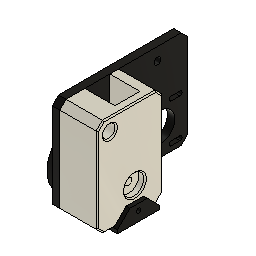
V2 Z Gearbox Buddy A (Autodesk Fusion 360 design; units mm, degrees)
Autodesk Fusion 360 part; units mm, degrees
sketch "Sketch1" plane through (0, 0, 0) normal (1, 0, 0) x (0, 1, 0)
  line L0 (21, 21) -> (-21, 21) construction
  line L1 (-21, 21) -> (-21, -21) construction
  line L2 (-21, -21) -> (21, -21) construction
  line L3 (21, -21) -> (21, 21) construction
  line L4 (21, 21) -> (-21, -21) construction
  line L5 (-21, 21) -> (21, -21) construction
  line L6 (15.5, 15.5) -> (-15.5, 15.5) construction
  line L7 (-15.5, 15.5) -> (-15.5, -15.5) construction
  line L8 (-15.5, -15.5) -> (15.5, -15.5) construction
  line L9 (15.5, -15.5) -> (15.5, 15.5) construction
  line L10 (15.5, 15.5) -> (-15.5, -15.5) construction
  line L11 (-15.5, 15.5) -> (15.5, -15.5) construction
  line L12 (21, -21) -> (-77, -21)
  line L13 (-77, -21) -> (-77, 57)
  line L14 (-77, 57) -> (21, 57)
  line L15 (21, 57) -> (21, -21) construction
  circle A0 centre (0, 0) radius 8 construction
  circle A1 centre (0, 0) radius 6.11 construction
  line L16 (-77, 37) -> (25, 37)
  line L17 (-77, 32) -> (25, 32)
  circle A2 centre (-47, 0) radius 30 construction
  circle A3 centre (0, 0) radius 2.75
  circle A4 centre (-47, 0) radius 2.75
  line L18 (-47, 37) -> (-47, 32)
  line L19 (19, 17.2) -> (12, 17.2)
  arc A5 (12, 17.2) -> (12, 13.8) centre (12, 15.5) ccw
  line L20 (12, 13.8) -> (19, 13.8)
  arc A6 (19, 13.8) -> (19, 17.2) centre (19, 15.5) ccw
  line L21 (19, 15.5) -> (12, 15.5) construction
  line L22 (-12, 17.2) -> (-19, 17.2)
  arc A7 (-19, 17.2) -> (-19, 13.8) centre (-19, 15.5) ccw
  arc A8 (-12, 13.8) -> (-12, 17.2) centre (-12, 15.5) ccw
  line L23 (-19, 13.8) -> (-12, 13.8)
  line L24 (19, -13.8) -> (12, -13.8)
  arc A9 (12, -13.8) -> (12, -17.2) centre (12, -15.5) ccw
  arc A10 (19, -17.2) -> (19, -13.8) centre (19, -15.5) ccw
  line L25 (12, -17.2) -> (19, -17.2)
  line L26 (-12, -13.8) -> (-19, -13.8)
  arc A11 (-19, -13.8) -> (-19, -17.2) centre (-19, -15.5) ccw
  arc A12 (-12, -17.2) -> (-12, -13.8) centre (-12, -15.5) ccw
  line L27 (-19, -17.2) -> (-12, -17.2)
  line L28 (21, 57) -> (25, 57)
  line L29 (25, 57) -> (25, -21)
  line L30 (25, -21) -> (21, -21)
  line L31 (21, -21) -> (21, 57) construction
  line L32 (-47, -21) -> (-47, 0) construction
  line L33 (-47, 0) -> (-77, 0) construction
  line L34 (0, 0) -> (-47, 0) construction
  point P0 (15.5, 15.5)
  dimension "d488" = 42
  dimension "d489" = 42
  dimension "d490" = 31
  dimension "d491" = 31
  dimension "d492" = 16
  dimension "d493" = 12.22
  dimension "d494" = 20
  dimension "d496" = 60
  dimension "d498" = 98
  dimension "d499" = 78
  dimension "d502" = 5.5
  dimension "d503" = 5.5
  dimension "d506" = 30
  dimension "d507" = 3.4
  dimension "d508" = 7
  dimension "d511" = -31
  dimension "d512" = -31
  dimension "d513" = 4
  dimension "d5757" = 30
  dimension "d5758" = 21
  dimension "d5762" = 102
  dimension "d5763" = 47
  constraint horizontal L0
  constraint perpendicular L0 L1
  constraint parallel L0 L2
  constraint parallel L1 L3
  constraint coincident L4 A0.centre
  constraint coincident L5 A0.centre
  constraint coincident A0.centre A1.centre
  constraint horizontal L6
  constraint perpendicular L6 L7
  constraint parallel L6 L8
  constraint parallel L7 L9
  constraint coincident L10 A0.centre
  constraint coincident L11 A0.centre
  constraint horizontal L12
  constraint vertical L13
  constraint horizontal L14
  constraint vertical L15
  constraint coincident L2.end L12
  constraint coincident L0.start L15
  constraint coincident L13 L16.start
  constraint perpendicular L13 L16
  constraint coincident L13 L17.start
  constraint concentric A2 A4
  constraint coincident L16 L18.start
  constraint coincident L17 L18.end
  constraint perpendicular L17 L18
  constraint tangent L19 A5
  constraint tangent A5 L20
  constraint parallel L19 L20
  constraint tangent L20 A6
  constraint tangent L19 A6
  constraint coincident L6 A5.centre
  constraint perpendicular L9 L21
  constraint coincident P0 L6.start
  constraint midpoint L21 P0
  constraint horizontal L28
  constraint vertical L29
  constraint horizontal L30
  constraint vertical L31
  constraint coincident L2.end L3.start
  constraint coincident L29 L16.end
  constraint coincident L29 L17.end
  constraint coincident L12 L32.start
  constraint perpendicular L12 L32
  constraint perpendicular L13 L33
  constraint coincident L13 L33.end
  constraint coincident A2.centre A4.centre
  measures "d488" distance of L0.start L2.end
  measures "d489" distance of L0.start L0.end
  measures "d490" distance of L7.end L8.end
  measures "d491" distance of L6.end L7.end
  measures "d492" diameter of A0
  measures "d493" diameter of A1
  measures "d494" distance of L14 L16
  measures "d496" diameter of A2
  measures "d498" distance of L2.end L12.end
  measures "d499" distance of L12.end L13.end
  measures "d502" diameter of A3
  measures "d503" diameter of A4
  measures "d506" distance of L13 L18
  measures "d507" diameter of A5
  measures "d508" distance of A6.centre A5.centre
  measures "d513" distance of L29.end L2.end
  measures "d5757" distance of L13 L32
  measures "d5758" distance of L12 L33
  measures "d5762" distance of L13 L29
  measures "d5763" distance of A2.centre A0.centre
extrude "Extrude1" add sketch "Sketch1" along normal blind 6 makes body 1
extrude "Extrude2" add sketch "Sketch1" against normal blind 20 contours L16 L17 L18 L29 bodies 1
sketch "Sketch2" plane through (0, 0, 0) normal (-1, 0, 0) x (0, -1, 0)
  line L0 (-25, 37) -> (47, 37)
  line L1 (47, 37) -> (47, 32)
  line L2 (47, 32) -> (-25, 32)
  line L3 (-25, 32) -> (-25, -21)
  line L4 (-25, -21) -> (77, -21)
  line L5 (77, -21) -> (77, 57)
  line L6 (77, 57) -> (-25, 57)
  line L7 (-25, 57) -> (-25, 37)
  line L8 (-12, -17.2) -> (-19, -17.2)
  arc A0 (-19, -13.8) -> (-19, -17.2) centre (-19, -15.5) ccw
  line L9 (-19, -13.8) -> (-12, -13.8)
  arc A1 (-12, -17.2) -> (-12, -13.8) centre (-12, -15.5) ccw
  arc A2 (-19, 17.2) -> (-19, 13.8) centre (-19, 15.5) ccw
  line L10 (-19, 17.2) -> (-12, 17.2)
  arc A3 (-12, 13.8) -> (-12, 17.2) centre (-12, 15.5) ccw
  line L11 (-12, 13.8) -> (-19, 13.8)
  line L12 (19, -17.2) -> (12, -17.2)
  arc A4 (12, -13.8) -> (12, -17.2) centre (12, -15.5) ccw
  line L13 (12, -13.8) -> (19, -13.8)
  arc A5 (19, -17.2) -> (19, -13.8) centre (19, -15.5) ccw
  line L14 (19, 13.8) -> (12, 13.8)
  arc A6 (12, 17.2) -> (12, 13.8) centre (12, 15.5) ccw
  line L15 (12, 17.2) -> (19, 17.2)
  arc A7 (19, 13.8) -> (19, 17.2) centre (19, 15.5) ccw
  circle A8 centre (47, 0) radius 2.75
  circle A9 centre (0, 0) radius 2.75
  line L16 (-3.5, -11.5) -> (3.5, -11.5)
  arc A10 (3.5, -11.5) -> (3.5, 11.5) centre (3.5, 0) ccw
  line L17 (3.5, 11.5) -> (-3.5, 11.5)
  arc A11 (-3.5, 11.5) -> (-3.5, -11.5) centre (-3.5, 0) ccw
  line L18 (-3.5, 0) -> (3.5, 0) construction
  line L19 (15.5, -15.5) -> (-15.5, -15.5) construction
  line L20 (-15.5, -15.5) -> (-15.5, 15.5) construction
  line L21 (-15.5, 15.5) -> (15.5, 15.5) construction
  line L22 (15.5, 15.5) -> (15.5, -15.5) construction
  line L23 (15.5, -15.5) -> (-15.5, 15.5) construction
  line L24 (-15.5, -15.5) -> (15.5, 15.5) construction
  line L25 (-18.5, 11.5) -> (-12.5, 11.5)
  arc A12 (-12.5, 11.5) -> (-12.5, 19.5) centre (-12.5, 15.5) ccw
  line L26 (-12.5, 19.5) -> (-18.5, 19.5)
  arc A13 (-18.5, 19.5) -> (-18.5, 11.5) centre (-18.5, 15.5) ccw
  line L27 (-18.5, 15.5) -> (-12.5, 15.5) construction
  line L28 (18.5, 19.5) -> (12.5, 19.5)
  arc A14 (12.5, 19.5) -> (12.5, 11.5) centre (12.5, 15.5) ccw
  arc A15 (18.5, 11.5) -> (18.5, 19.5) centre (18.5, 15.5) ccw
  line L29 (12.5, 11.5) -> (18.5, 11.5)
  line L30 (-12.5, -11.5) -> (-18.5, -11.5)
  arc A16 (-18.5, -11.5) -> (-18.5, -19.5) centre (-18.5, -15.5) ccw
  arc A17 (-12.5, -19.5) -> (-12.5, -11.5) centre (-12.5, -15.5) ccw
  line L31 (-18.5, -19.5) -> (-12.5, -19.5)
  line L32 (18.5, -11.5) -> (12.5, -11.5)
  arc A18 (12.5, -11.5) -> (12.5, -19.5) centre (12.5, -15.5) ccw
  arc A19 (18.5, -19.5) -> (18.5, -11.5) centre (18.5, -15.5) ccw
  line L33 (12.5, -19.5) -> (18.5, -19.5)
  point P0 (-15.5, 15.5)
  dimension "d514" = 23
  dimension "d515" = 7
  dimension "d556" = 31
  dimension "d557" = 31
  dimension "d558" = 4
  dimension "d559" = 6
  dimension "d562" = 31
  dimension "d563" = -31
  constraint tangent L16 A10
  constraint tangent A10 L17
  constraint parallel L16 L17
  constraint tangent L17 A11
  constraint tangent L16 A11
  constraint perpendicular L3 L18
  constraint coincident A9.centre origin
  constraint midpoint L18 A9.centre
  constraint horizontal L19
  constraint perpendicular L19 L20
  constraint parallel L19 L21
  constraint parallel L20 L22
  constraint coincident L23 A9.centre
  constraint coincident L24 A9.centre
  constraint tangent L25 A12
  constraint tangent A12 L26
  constraint parallel L25 L26
  constraint tangent L26 A13
  constraint tangent L25 A13
  constraint coincident L21 A12.centre
  constraint perpendicular L20 L27
  constraint coincident P0 L20.end
  constraint midpoint L27 P0
  measures "d514" diameter of A10
  measures "d515" distance of A11.centre A10.centre
  measures "d556" distance of P0 L21.end
  measures "d557" distance of L19.end P0
  measures "d558" radius of A12
  measures "d559" distance of A13.centre A12.centre
extrude "Extrude3" cut sketch "Sketch2" against normal through all contours L16 A10 L17 A11 bodies 1
extrude "Extrude4" cut sketch "Sketch2" against normal blind 1.5 contours L25 A12 L26 A13 | L28 A14 A15 L29 | L30 A16 A17 L31 | L32 A18 A19 L33 bodies 1
hole "Hole1" at (-10, -11, 37) direction (0, 0, -1) diameter 5.5 end through all bodies 1
sketch "Sketch3" plane through (0, 0, 0) normal (-1, 0, 0) x (0, -1, 0)
  line L0 (-3.5, 11.5) -> (3.5, 11.5)
  arc A0 (3.5, -11.5) -> (3.5, 11.5) centre (3.5, 0) ccw
  line L1 (3.5, -11.5) -> (-3.5, -11.5)
  arc A1 (-3.5, 11.5) -> (-3.5, -11.5) centre (-3.5, 0) ccw
  line L2 (-25, 37) -> (47, 37)
  line L3 (47, 37) -> (47, 32)
  line L4 (47, 32) -> (-25, 32)
  line L5 (-25, 32) -> (-25, -21)
  line L6 (-25, -21) -> (77, -21)
  line L7 (77, -21) -> (77, 57)
  line L8 (77, 57) -> (-25, 57)
  line L9 (-25, 57) -> (-25, 37)
  circle A2 centre (47, 0) radius 2.75
  line L10 (-25, 57) -> (-25, 37)
  line L11 (-25, 47) -> (-1, 47) construction
  arc A3 (18.5, 11.5) -> (18.5, 19.5) centre (18.5, 15.5) ccw
  line L12 (18.5, 11.5) -> (12.5, 11.5)
  arc A4 (12.5, 19.5) -> (12.5, 11.5) centre (12.5, 15.5) ccw
  line L13 (12.5, 19.5) -> (18.5, 19.5)
  arc A5 (18.5, -19.5) -> (18.5, -11.5) centre (18.5, -15.5) ccw
  line L14 (18.5, -19.5) -> (12.5, -19.5)
  arc A6 (12.5, -11.5) -> (12.5, -19.5) centre (12.5, -15.5) ccw
  line L15 (12.5, -11.5) -> (18.5, -11.5)
  line L16 (-12.5, 11.5) -> (-18.5, 11.5)
  arc A7 (-18.5, 19.5) -> (-18.5, 11.5) centre (-18.5, 15.5) ccw
  line L17 (-18.5, 19.5) -> (-12.5, 19.5)
  arc A8 (-12.5, 11.5) -> (-12.5, 19.5) centre (-12.5, 15.5) ccw
  arc A9 (-12.5, -19.5) -> (-12.5, -11.5) centre (-12.5, -15.5) ccw
  line L18 (-12.5, -19.5) -> (-18.5, -19.5)
  arc A10 (-18.5, -11.5) -> (-18.5, -19.5) centre (-18.5, -15.5) ccw
  line L19 (-18.5, -11.5) -> (-12.5, -11.5)
  dimension "d549" = 24
  constraint midpoint L10 L11.start
  constraint perpendicular L10 L11
  measures "d549" distance of L11.start L11.end
hole "Hole3" at (0, 1, 47) direction (1, 0, 0) diameter 5.5 end through all bodies 1
hole "Hole4" at (0, -47, 0) direction (1, 0, 0) diameter 16.2 depth 5 tip angle 180 bodies 1
chamfer "Chamfer1" distance 20 angle 45 2 edges at (-20, 25, 34.5) (-20, -47, 34.5) on bodies 1
chamfer "Chamfer2" distance 5 angle 45 4 edges at (3, -77, 57) (3, -77, -21) (3, 25, -21) (3, 25, 57) on bodies 1
chamfer "Chamfer3" distance 0.5 angle 45 1 edges at (0, -39.4481, 2.9291) on bodies 1
sketch "Sketch1 (2)" plane through (6, 0, 0) normal (1, 0, 0) x (0, 1, 0) in component "V2 Z Gearbox Cover A"
  line L0 (25, 52) -> (20, 57)
  line L1 (20, 57) -> (-72, 57)
  line L2 (-72, 57) -> (-77, 52)
  line L3 (-77, 52) -> (-77, -16)
  line L4 (-77, -16) -> (-72, -21)
  line L5 (-72, -21) -> (20, -21)
  line L6 (20, -21) -> (25, -16)
  line L7 (25, -16) -> (25, 52)
  line L8 (-3.5, 11.5) -> (3.5, 11.5)
  arc A0 (3.5, -11.5) -> (3.5, 11.5) centre (3.5, 0) ccw
  line L9 (3.5, -11.5) -> (-3.5, -11.5)
  arc A1 (-3.5, 11.5) -> (-3.5, -11.5) centre (-3.5, 0) ccw
  line L10 (19, -17.2) -> (12, -17.2)
  arc A2 (12, -13.8) -> (12, -17.2) centre (12, -15.5) ccw
  line L11 (12, -13.8) -> (19, -13.8)
  arc A3 (19, -17.2) -> (19, -13.8) centre (19, -15.5) ccw
  line L12 (-12, -17.2) -> (-19, -17.2)
  arc A4 (-19, -13.8) -> (-19, -17.2) centre (-19, -15.5) ccw
  line L13 (-19, -13.8) -> (-12, -13.8)
  arc A5 (-12, -17.2) -> (-12, -13.8) centre (-12, -15.5) ccw
  circle A6 centre (-47, 0) radius 2.75
  arc A7 (19, 13.8) -> (19, 17.2) centre (19, 15.5) ccw
  line L14 (19, 13.8) -> (12, 13.8)
  arc A8 (12, 17.2) -> (12, 13.8) centre (12, 15.5) ccw
  line L15 (12, 17.2) -> (19, 17.2)
  line L16 (-12, 13.8) -> (-19, 13.8)
  arc A9 (-19, 17.2) -> (-19, 13.8) centre (-19, 15.5) ccw
  line L17 (-19, 17.2) -> (-12, 17.2)
  arc A10 (-12, 13.8) -> (-12, 17.2) centre (-12, 15.5) ccw
  circle A11 centre (-47, 0) radius 2.75
  line L18 (-47, 0) -> (-47, 57) construction
  line L19 (-47, 32) -> (25, 32)
  line L20 (21, -21) -> (-21, -21) construction
  line L21 (-21, -21) -> (-21, 21) construction
  line L22 (-21, 21) -> (21, 21) construction
  line L23 (21, 21) -> (21, -21) construction
  line L24 (21, -21) -> (-21, 21) construction
  line L25 (-21, -21) -> (21, 21) construction
  line L26 (-69, 57) -> (-25, 57)
  line L27 (-25, 57) -> (-25, -21)
  line L28 (-25, -21) -> (-69, -21)
  line L29 (-69, -21) -> (-69, 57)
  circle A12 centre (1, 47) radius 2.75
  point P0 (-47, 57)
  dimension "d521" = 42
  dimension "d522" = 42
  dimension "d524" = 44
  dimension "d525" = 4
  constraint coincident A6.centre A11.centre
  constraint perpendicular L1 L18
  constraint coincident P0 L18.end
  constraint horizontal L20
  constraint perpendicular L20 L21
  constraint parallel L20 L22
  constraint parallel L21 L23
  constraint coincident L24 origin
  constraint coincident L25 origin
  constraint horizontal L26
  constraint vertical L27
  constraint horizontal L28
  constraint vertical L29
  constraint coincident L5 L27.end
  constraint midpoint P0 L26
  constraint coincident L1 L26.start
  measures "d521" distance of L21.end L22.end
  measures "d522" distance of L20.end L21.end
  measures "d524" distance of L27.end L28.end
  measures "d525" distance of L21 L27
extrude "Extrude1'" add sketch "Sketch1 (2)" along normal blind 30 separate body contours L1 L5 L26 L27 L28 L29 makes body 2 in component "V2 Z Gearbox Cover A"
sketch "Sketch2 (2)" plane through (0, 0, 57) normal (0, 0, 1) x (-1, 0, 0) in component "V2 Z Gearbox Cover A"
  line L0 (-36, 44.25) -> (-36, 49.75)
  line L1 (-6, 44.25) -> (-6, 49.75)
  line L2 (-6, 47) -> (-18, 47) construction
  line L3 (-6, 57) -> (-30, 57)
  line L4 (-30, 57) -> (-30, 37)
  line L5 (-30, 37) -> (-6, 37)
  line L6 (-6, 37) -> (-6, 57)
  line L7 (-6, 57) -> (-30, 37) construction
  line L8 (-30, 57) -> (-6, 37) construction
  line L9 (-6, 69) -> (-6, 25)
  point P0 (-18, 47)
  dimension "d528" = 20
  dimension "d529" = 24
  dimension "d530" = 6
  constraint midpoint L1 L2.start
  constraint perpendicular L1 L2
  constraint horizontal L3
  constraint perpendicular L3 L4
  constraint parallel L3 L5
  constraint parallel L4 L6
  constraint coincident L7 P0
  constraint coincident L8 P0
  constraint coincident P0 L2.end
  constraint coincident L3.start L9
  measures "d528" distance of L3.end L4.end
  measures "d529" distance of L4 L6
  measures "d530" distance of L0 L4
extrude "Extrude2'" cut sketch "Sketch2 (2)" against normal through all bodies 2 in component "V2 Z Gearbox Cover A"
extrude "Extrude3'" add 1 faces at (16, -69, 5) along direction (0, -1, 0) up to surface (8 mm away) on bodies 2 bodies 2 in component "V2 Z Gearbox Cover A"
hole "Hole1'" at (36, -47, 0) direction (-1, 0, 0) diameter 16.2 depth 5 tip angle 180 bodies 2 in component "V2 Z Gearbox Cover A"
sketch "Sketch3 (2)" plane through (36, 0, 0) normal (1, 0, 0) x (0, 1, 0) in component "V2 Z Gearbox Cover A"
  line L0 (-77, 57) -> (-57, 57)
  line L1 (-67, 57) -> (-67, 47) construction
  dimension "d546" = 10
  constraint midpoint L0 L1.start
  constraint perpendicular L0 L1
  measures "d546" distance of L1.start L1.end
hole "Hole2" at (36, -67, 47) direction (-1, 0, 0) diameter 5.5 end through all counterbore diameter 10 counterbore depth 21 bodies 1
hole "Hole2'" at (36, -67, 47) direction (-1, 0, 0) diameter 5.5 end through all counterbore diameter 10 counterbore depth 21 bodies 1 2 in component "V2 Z Gearbox Cover A"
sketch "Sketch4" plane through (31, 0, 0) normal (1, 0, 0) x (0, 1, 0) in component "V2 Z Gearbox Cover A"
  circle A0 centre (-47, 0) radius 2.75
  circle A1 centre (-47, 0) radius 8.1
  circle A2 centre (-47, 0) radius 2.75
extrude "Extrude4'" add sketch "Sketch4" against normal blind 0.3 contours A0 A2 bodies 2 in component "V2 Z Gearbox Cover A"
sketch "Sketch5" plane through (15, 0, 0) normal (1, 0, 0) x (0, 1, 0) in component "V2 Z Gearbox Cover A"
  circle A0 centre (-67, 47) radius 5
  circle A1 centre (-67, 47) radius 2.75
  circle A2 centre (-67, 47) radius 2.75
extrude "Extrude5" add sketch "Sketch5" against normal blind 0.3 contours A1 A2 bodies 2 in component "V2 Z Gearbox Cover A"
chamfer "Chamfer1'" distance 5 angle 45 4 edges at (21, -77, 57) (21, -25, 57) (21, -77, -21) (21, -25, -21) on bodies 2 in component "V2 Z Gearbox Cover A"
chamfer "Chamfer2'" distance 1 angle 45 1 faces at (36, -44.4875, 34.8365) on bodies 2 in component "V2 Z Gearbox Cover A"
sketch "Sketch6" plane through (36, 0, 0) normal (1, 0, 0) x (0, 1, 0) in component "V2 Z Gearbox Cover A"
  circle A0 centre (-67, 47) radius 6
  line L0 (-71.5858, -20) -> (-30.4142, -20)
  line L1 (-30.4142, -20) -> (-26, -15.5858)
  line L2 (-26, -15.5858) -> (-26, 51.5858)
  line L3 (-26, 51.5858) -> (-30.4142, 56)
  line L4 (-30.4142, 56) -> (-71.5858, 56)
  line L5 (-71.5858, 56) -> (-76, 51.5858)
  line L6 (-76, 51.5858) -> (-76, -15.5858)
  line L7 (-76, -15.5858) -> (-71.5858, -20)
  circle A1 centre (-47, 0) radius 9.1
  line L8 (-57, -21) -> (-37, -21)
  line L9 (-47, -21) -> (-47, -11) construction
  circle A2 centre (-47, -16) radius 1.25 construction
  dimension "d6087" = 10
  dimension "d6088" = 2.5
  constraint midpoint L8 L9.start
  constraint perpendicular L0 L9
  constraint midpoint L9 A2.centre
  measures "d6087" distance of L9.start L9.end
  measures "d6088" diameter of A2
hole "Hole3'" at (36, -47, -16) direction (-1, 0, 0) diameter 2.529 depth 16 tip angle 118 bodies 2 in component "V2 Z Gearbox Cover A"
thread "Thread1" "ISO Metric profile 3.0 M3x0.5 M3x0.5 6H" major diameter 3.086 minor diameter 2.529 pitch 0.5 angle 60 resizes the face on face at (34, -47.8128, -16.9687) on bodies 2 in component "V2 Z Gearbox Cover A"
sketch "Sketch1 (3)" plane through (0, 0, -21) normal (0, 0, -1) x (1, 0, 0) in component "V2 Z Gearbox Dust Cover AB"
  line L0 (6, 57) -> (30, 57)
  line L1 (30, 57) -> (30, 37)
  line L2 (30, 37) -> (6, 37)
  line L3 (6, 72) -> (6, -20)
  line L4 (35, 30) -> (6, 30)
  line L5 (36, 30.4142) -> (36, 71.5858)
  line L6 (6, 47) -> (36, 47) construction
  line L7 (36, 30) -> (6, 30)
  line L8 (6, 30) -> (6, 64)
  line L9 (6, 64) -> (36, 64)
  line L10 (36, 64) -> (36, 30)
  line L11 (36, 30) -> (6, 64) construction
  line L12 (6, 30) -> (36, 64) construction
  point P0 (30, 47)
  point P1 (21, 47)
  constraint coincident L3 L6.start
  constraint coincident L5 L6.end
  constraint perpendicular L5 L6
  constraint coincident L6 P0
  constraint midpoint L1 P0
  constraint horizontal L7
  constraint perpendicular L7 L8
  constraint parallel L7 L9
  constraint parallel L8 L10
  constraint coincident L11 P1
  constraint coincident L12 P1
  constraint coincident L6 P1
  constraint coincident L5 L9.end
  constraint coincident L3 L8.end
  constraint coincident L4.end L7.end
extrude "Extrude1''" add sketch "Sketch1 (3)" along normal blind 3 separate body makes body 3 in component "V2 Z Gearbox Dust Cover AB"
sketch "Sketch2 (3)" plane through (0, 0, -21) normal (0, 0, 1) x (-1, 0, 0) in component "V2 Z Gearbox Dust Cover AB"
  line L0 (-35, 72) -> (-35, 30)
  line L1 (-35, 30) -> (-6, 30)
  line L2 (-6, 30) -> (-6, 37)
  line L3 (-6, 37) -> (-30, 37)
  line L4 (-30, 37) -> (-30, 57)
  line L5 (-30, 57) -> (-6, 57)
  line L6 (-6, 57) -> (-6, 72)
  line L7 (-6, 72) -> (-35, 72)
  line L8 (-6, 37) -> (-6, 57)
  line L9 (-6, 64) -> (-36, 64)
  line L10 (-36, 64) -> (-36, 30)
  line L11 (-36, 30) -> (-6, 30)
  line L12 (-6, 30) -> (-6, 64)
  constraint coincident L2.end L3.start
  constraint coincident L5.end L6.start
extrude "Extrude2''" add sketch "Sketch2 (3)" along normal blind 4 thin wall 2 on the right open curves L8 L3 L4 L5 bodies 3 in component "V2 Z Gearbox Dust Cover AB"
sketch "Sketch3 (3)" plane through (36, 0, 0) normal (1, 0, 0) x (0, 1, 0) in component "V2 Z Gearbox Dust Cover AB"
  line L0 (-30, -21) -> (-64, -21)
  line L1 (-64, -21) -> (-64, -24)
  line L2 (-64, -24) -> (-30, -24)
  line L3 (-30, -24) -> (-30, -21)
  line L4 (-64, -24) -> (-30, -24)
  line L5 (-30, -24) -> (-30, -11)
  line L6 (-30, -11) -> (-64, -11)
  line L7 (-64, -11) -> (-64, -24)
  line L8 (-47, -11) -> (-47, -21) construction
  circle A0 centre (-47, -16) radius 1.75
  dimension "d6079" = 13
  dimension "d6080" = 3.5
  constraint horizontal L4
  constraint vertical L5
  constraint horizontal L6
  constraint vertical L7
  constraint coincident L1.end L2.start
  constraint coincident L2.end L3.start
  constraint midpoint L6 L8.start
  constraint midpoint L0 L8.end
  constraint midpoint L8 A0.centre
  measures "d6079" distance of L2.end L5.end
  measures "d6080" diameter of A0
extrude "Extrude3''" add sketch "Sketch3 (3)" along normal blind 3 bodies 3 in component "V2 Z Gearbox Dust Cover AB"
fillet "Fillet1" radius 4 2 edges at (6, -64, -22.5) (6, -30, -22.5) on bodies 3 in component "V2 Z Gearbox Dust Cover AB"
chamfer "Chamfer1''" distance 10 angle 45 2 edges at (37.5, -64, -11) (37.5, -30, -11) on bodies 3 in component "V2 Z Gearbox Dust Cover AB"
chamfer "Chamfer1''" distance 0.3 angle 45 1 faces at (19.6667, -41.3333, -24) on bodies 3 in component "V2 Z Gearbox Dust Cover AB"
sketch "Sketch1 (4)" plane through (0, 0, 0) normal (-1, 0, 0) x (0, -1, 0) in component "V2 Gearbox Belt ABC"
  circle A0 centre (67, 47) radius 2.75
  circle A1 centre (-1, 47) radius 2.75
  circle A2 centre (47, 0) radius 8.6
  circle A3 centre (0, 0) radius 6.11 construction
  circle A4 centre (47, 0) radius 25.25 construction
  line L0 (-2.4882, 5.5804) -> (36.7173, 23.0614)
  line L1 (-2.4882, -5.5804) -> (36.7173, -23.0614)
  arc A5 (-2.4882, 5.5804) -> (-2.4882, -5.5804) centre (0, 0) ccw
  arc A6 (36.7173, -23.0614) -> (36.7173, 23.0614) centre (47, 0) ccw
  dimension "d3110" = 12.22
  dimension "d3111" = 50.5
  constraint coincident A3.centre A5.centre
  constraint concentric A2 A4
  constraint coincident A3 L0.start
  constraint coincident A4 L0.end
  constraint coincident A3 L1.start
  constraint coincident A4 L1.end
  constraint tangent A4 L0
  constraint tangent A3 L0
  constraint tangent A3 L1
  constraint tangent A4 L1
  constraint tangent L0 A5
  constraint tangent L1 A6
  measures "d3110" diameter of A3
  measures "d3111" diameter of A4
extrude "Extrude1'''" add sketch "Sketch1 (4)" along normal blind 6 from surface at 3 thin wall 1 on the right separate body open curves A6 L1 A5 L0 makes body 4 in component "V2 Gearbox Belt ABC"
component "V2 Z Gearbox Cover A" placed x (1, 0, 0) y (0, 1, 0) z (0, 0, 1) at (0, 0, 0)
component "V2 Z Gearbox Dust Cover AB" placed x (1, 0, 0) y (0, 1, 0) z (0, 0, 1) at (0, 0, 0)
component "V2 Gearbox Belt ABC" placed x (1, 0, 0) y (0, 1, 0) z (0, 0, 1) at (0, 0, 0)
named bodies: "V2 Z Gearbox Buddy A_1x", "V2 Z Gearbox Cover A_1x", "V2 Z Gearbox Dust Cover AB_2x"
